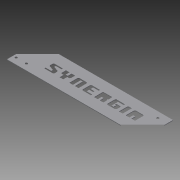
# Autodesk Inventor part: logo
Saved by Autodesk Inventor 2015 SP1 (Build 190203100, 203)
## iProperties
Created: 2015-04-17
Part Number: logo
Material: Ogólny
Document SubType Name: Konstrukcja blachowa
Designer: Marcin
Density: 1 g/cm^3
Appearance: Domyślna
Sheet Metal Rule: Domyślny
Author: Marcin
Autodesk Inventor part; units mm, degrees
ref_plane "YZ Plane" through (0, 0, 0) normal (1, 0, 0) x (0, 1, 0)
ref_plane "XZ Plane" through (0, 0, 0) normal (0, 1, 0) x (-1, 0, 0)
ref_plane "XY Plane" through (0, 0, 0) normal (0, 0, 1) x (1, 0, 0)
sketch "Szkic3" plane through (0, 0, 0) normal (0, 0, 1) x (1, 0, 0)
  line L0 (-89, -20) -> (89, -20)
  line L1 (89, -20) -> (89, 20)
  line L2 (89, 20) -> (-89, 20)
  line L3 (-89, 20) -> (-89, -20)
  line L4 (-89, -20) -> (89, 20) construction
  line L5 (89, -20) -> (-89, 20) construction
  point P0 (0, 0)
  dimension "d3" = 40
  dimension "d4" = 178
  measures "d3" distance of L0.end L1.end
  measures "d4" distance of L1.end L2.end
extrude "Płyta1" add sketch "Szkic3" along normal blind 0.8
sketch "Blok1" plane through (0, 0, 0) normal (0, 0, 1) x (1, 0, 0)
  line L0 (194.8054, -79.0716) -> (189.6563, -79.0716)
  line L1 (189.6563, -79.0716) -> (189.6563, -80.7591)
  line L2 (189.6563, -80.7591) -> (191.2238, -80.7591)
  line L3 (191.2238, -80.7591) -> (191.2238, -84.2418)
  line L4 (191.2238, -84.2418) -> (188.4658, -84.2418)
  line L5 (188.4658, -84.2418) -> (188.4658, -75.6126)
  line L6 (199.9976, -85.9056) -> (204.832, -85.9056)
  line L7 (204.832, -85.9056) -> (204.832, -73.9056)
  line L8 (204.832, -73.9056) -> (201.1445, -73.9056)
  line L9 (199.9976, -85.9056) -> (199.9976, -75.0767)
  line L10 (199.9976, -75.0767) -> (201.1445, -73.9056)
  line L11 (208.9177, -85.9056) -> (213.7175, -85.9056)
  line L12 (213.7175, -85.9056) -> (213.7175, -80.7591)
  line L13 (213.7175, -80.7591) -> (216.4159, -80.7591)
  line L14 (216.4159, -80.7591) -> (216.4159, -85.9056)
  line L15 (216.4159, -85.9056) -> (221.086, -85.9056)
  line L16 (221.086, -85.9056) -> (221.086, -75.0767)
  line L17 (221.086, -75.0767) -> (220.0494, -73.9056)
  line L18 (220.0494, -73.9056) -> (210.0722, -73.9056)
  line L19 (210.0722, -73.9056) -> (208.9177, -75.0767)
  line L20 (208.9177, -75.0767) -> (208.9177, -85.9056)
  line L21 (213.6195, -79.0716) -> (216.4159, -79.0716)
  line L22 (216.4159, -79.0716) -> (216.4159, -75.6126)
  line L23 (216.4159, -75.6126) -> (213.7175, -75.6126)
  line L24 (213.7175, -75.6126) -> (213.6195, -75.6126)
  line L25 (213.6195, -75.6126) -> (213.6195, -79.0716)
  line L26 (188.4658, -75.6126) -> (195.9066, -75.6126)
  line L27 (102.1862, -84.2418) -> (102.1862, -85.9056)
  line L28 (102.1862, -85.9056) -> (113.4232, -85.9056)
  line L29 (113.4232, -85.9056) -> (114.3485, -84.8496)
  line L30 (114.3485, -84.8496) -> (114.3485, -81.0367)
  line L31 (114.3485, -81.0367) -> (113.5668, -80.0795)
  line L32 (113.5668, -80.0795) -> (106.7866, -77.6387)
  line L33 (106.7866, -77.6387) -> (106.7866, -75.6126)
  line L34 (106.7866, -75.6126) -> (114.3485, -75.6126)
  line L35 (114.3485, -75.6126) -> (114.3485, -73.9056)
  line L36 (114.3485, -73.9056) -> (103.2928, -73.9056)
  line L37 (103.2928, -73.9056) -> (102.3186, -75.0175)
  line L38 (102.3186, -75.0175) -> (102.1862, -78.6916)
  line L39 (102.1862, -78.6916) -> (103.0668, -79.7699)
  line L40 (103.0668, -79.7699) -> (109.5514, -82.1043)
  line L41 (109.5514, -82.1043) -> (109.5514, -84.2418)
  line L42 (109.5514, -84.2418) -> (102.1862, -84.2418)
  line L43 (118.5153, -73.9056) -> (118.5153, -79.3691)
  line L44 (118.5153, -79.3691) -> (119.5796, -80.6723)
  line L45 (119.5796, -80.6723) -> (122.2512, -80.6723)
  line L46 (122.2512, -80.6723) -> (122.2512, -85.9056)
  line L47 (122.2512, -85.9056) -> (126.8723, -85.9056)
  line L48 (126.8723, -85.9056) -> (126.8723, -80.6723)
  line L49 (126.8723, -80.6723) -> (129.6451, -80.6723)
  line L50 (129.6451, -80.6723) -> (130.5602, -79.6279)
  line L51 (130.5602, -79.6279) -> (130.5602, -73.9056)
  line L52 (130.5602, -73.9056) -> (125.9666, -73.9056)
  line L53 (125.9666, -73.9056) -> (125.9666, -79.0339)
  line L54 (125.9666, -79.0339) -> (123.1426, -79.0339)
  line L55 (123.1426, -79.0339) -> (123.1426, -73.9056)
  line L56 (123.1426, -73.9056) -> (118.5153, -73.9056)
  line L57 (134.8965, -85.9056) -> (139.482, -85.9056)
  line L58 (139.482, -85.9056) -> (139.482, -75.6126)
  line L59 (139.482, -75.6126) -> (142.2406, -75.6126)
  line L60 (142.2406, -75.6126) -> (142.2406, -85.9056)
  line L61 (142.2406, -85.9056) -> (146.9336, -85.9056)
  line L62 (146.9336, -85.9056) -> (146.9336, -75.2319)
  line L63 (146.9336, -75.2319) -> (145.8504, -73.9056)
  line L64 (145.8504, -73.9056) -> (136.007, -73.9056)
  line L65 (136.007, -73.9056) -> (134.8965, -75.1731)
  line L66 (134.8965, -75.1731) -> (134.8965, -85.9056)
  line L67 (163.2215, -85.9056) -> (163.2215, -84.2418)
  line L68 (163.2215, -84.2418) -> (155.8113, -84.2418)
  line L69 (155.8113, -84.2418) -> (155.8113, -80.7591)
  line L70 (155.8113, -80.7591) -> (160.8725, -80.7591)
  line L71 (160.8725, -80.7591) -> (160.8725, -79.0339)
  line L72 (160.8725, -79.0339) -> (155.8113, -79.0339)
  line L73 (155.8113, -79.0339) -> (155.8113, -75.6126)
  line L74 (155.8113, -75.6126) -> (163.2215, -75.6126)
  line L75 (163.2215, -75.6126) -> (163.2215, -73.9056)
  line L76 (163.2215, -73.9056) -> (152.3241, -73.9056)
  line L77 (152.3241, -73.9056) -> (151.2136, -75.1731)
  line L78 (151.2136, -75.1731) -> (151.2136, -84.8496)
  line L79 (151.2136, -84.8496) -> (152.3241, -85.9056)
  line L80 (152.3241, -85.9056) -> (163.2215, -85.9056)
  line L81 (167.3998, -85.9056) -> (172.1189, -85.9056)
  line L82 (172.1189, -85.9056) -> (172.1189, -80.6723)
  line L83 (172.1189, -80.6723) -> (174.8793, -80.6723)
  line L84 (174.8793, -80.6723) -> (174.8793, -85.9056)
  line L85 (174.8793, -85.9056) -> (179.5438, -85.9056)
  line L86 (179.5438, -85.9056) -> (179.5438, -81.0367)
  line L87 (179.5438, -81.0367) -> (178.6965, -80.0795)
  line L88 (178.6965, -80.0795) -> (178.6965, -79.8231)
  line L89 (178.6965, -79.8231) -> (179.5438, -78.9321)
  line L90 (179.5438, -78.9321) -> (179.5438, -75.0767)
  line L91 (179.5438, -75.0767) -> (178.4192, -74.0073)
  line L92 (178.4192, -74.0073) -> (168.5273, -74.0834)
  line L93 (168.5273, -74.0834) -> (167.3998, -75.2692)
  line L94 (167.3998, -75.2692) -> (167.3998, -85.9056)
  line L95 (172.1189, -75.6126) -> (172.1189, -79.0339)
  line L96 (172.1189, -79.0339) -> (174.8793, -79.0339)
  line L97 (174.8793, -79.0339) -> (174.8793, -75.6126)
  line L98 (174.8793, -75.6126) -> (172.1189, -75.6126)
  line L99 (195.9066, -75.6126) -> (195.9066, -73.9056)
  line L100 (195.9066, -73.9056) -> (184.8247, -73.9056)
  line L101 (184.8247, -73.9056) -> (183.7111, -75.0767)
  line L102 (183.7111, -75.0767) -> (183.7111, -84.7811)
  line L103 (183.7111, -84.7811) -> (184.7064, -85.9056)
  line L104 (184.7064, -85.9056) -> (194.8054, -85.9056)
  line L105 (194.8054, -85.9056) -> (195.9066, -84.7811)
  line L106 (195.9066, -84.7811) -> (195.9066, -80.1501)
  line L107 (195.9066, -80.1501) -> (194.8054, -79.0716)
  point P0 (162.2151, -79.6004)
  dimension "d0" = 12
  measures "d0" distance between parallel lines of L36 L28
sketch "Szkic4" plane through (0, 0, 0.8) normal (0, 0, 1) x (1, 0, 0)
  line L0 (-89, -20) -> (-89, 20) projected
  line L1 (38.5569, 1.0581) -> (33.4078, 1.0581)
  line L2 (33.4078, 1.0581) -> (33.4078, -0.6294)
  line L3 (33.4078, -0.6294) -> (34.9753, -0.6294)
  line L4 (34.9753, -0.6294) -> (34.9753, -4.1121)
  line L5 (34.9753, -4.1121) -> (32.2172, -4.1121)
  line L6 (32.2172, -4.1121) -> (32.2172, 4.5171)
  line L7 (43.7491, -5.7759) -> (48.5835, -5.7759)
  line L8 (48.5835, -5.7759) -> (48.5835, 6.2241)
  line L9 (48.5835, 6.2241) -> (44.8959, 6.2241)
  line L10 (43.7491, -5.7759) -> (43.7491, 5.053)
  line L11 (43.7491, 5.053) -> (44.8959, 6.2241)
  line L12 (52.6692, -5.7759) -> (57.469, -5.7759)
  line L13 (57.469, -5.7759) -> (57.469, -0.6294)
  line L14 (57.469, -0.6294) -> (60.1673, -0.6294)
  line L15 (60.1673, -0.6294) -> (60.1673, -5.7759)
  line L16 (60.1673, -5.7759) -> (64.8375, -5.7759)
  line L17 (64.8375, -5.7759) -> (64.8375, 5.053)
  line L18 (64.8375, 5.053) -> (63.8009, 6.2241)
  line L19 (63.8009, 6.2241) -> (53.8237, 6.2241)
  line L20 (53.8237, 6.2241) -> (52.6692, 5.053)
  line L21 (52.6692, 5.053) -> (52.6692, -5.7759)
  line L22 (57.371, 1.0581) -> (60.1673, 1.0581)
  line L23 (60.1673, 1.0581) -> (60.1673, 4.5171)
  line L24 (60.1673, 4.5171) -> (57.469, 4.5171)
  line L25 (57.469, 4.5171) -> (57.371, 4.5171)
  line L26 (57.371, 4.5171) -> (57.371, 1.0581)
  line L27 (32.2172, 4.5171) -> (39.6581, 4.5171)
  line L28 (-54.0623, -4.1121) -> (-54.0623, -5.7759)
  line L29 (-54.0623, -5.7759) -> (-42.8254, -5.7759)
  line L30 (-42.8254, -5.7759) -> (-41.9001, -4.7199)
  line L31 (-41.9001, -4.7199) -> (-41.9001, -0.9071)
  line L32 (-41.9001, -0.9071) -> (-42.6818, 0.0501)
  line L33 (-42.6818, 0.0501) -> (-49.4619, 2.491)
  line L34 (-49.4619, 2.491) -> (-49.4619, 4.5171)
  line L35 (-49.4619, 4.5171) -> (-41.9001, 4.5171)
  line L36 (-41.9001, 4.5171) -> (-41.9001, 6.2241)
  line L37 (-41.9001, 6.2241) -> (-52.9557, 6.2241)
  line L38 (-52.9557, 6.2241) -> (-53.9299, 5.1122)
  line L39 (-53.9299, 5.1122) -> (-54.0623, 1.4381)
  line L40 (-54.0623, 1.4381) -> (-53.1817, 0.3598)
  line L41 (-53.1817, 0.3598) -> (-46.6971, -1.9747)
  line L42 (-46.6971, -1.9747) -> (-46.6971, -4.1121)
  line L43 (-46.6971, -4.1121) -> (-54.0623, -4.1121)
  line L44 (-37.7332, 6.2241) -> (-37.7332, 0.7606)
  line L45 (-37.7332, 0.7606) -> (-36.6689, -0.5426)
  line L46 (-36.6689, -0.5426) -> (-33.9974, -0.5426)
  line L47 (-33.9974, -0.5426) -> (-33.9974, -5.7759)
  line L48 (-33.9974, -5.7759) -> (-29.3763, -5.7759)
  line L49 (-29.3763, -5.7759) -> (-29.3763, -0.5426)
  line L50 (-29.3763, -0.5426) -> (-26.6034, -0.5426)
  line L51 (-26.6034, -0.5426) -> (-25.6884, 0.5017)
  line L52 (-25.6884, 0.5017) -> (-25.6884, 6.2241)
  line L53 (-25.6884, 6.2241) -> (-30.282, 6.2241)
  line L54 (-30.282, 6.2241) -> (-30.282, 1.0958)
  line L55 (-30.282, 1.0958) -> (-33.1059, 1.0958)
  line L56 (-33.1059, 1.0958) -> (-33.1059, 6.2241)
  line L57 (-33.1059, 6.2241) -> (-37.7332, 6.2241)
  line L58 (-21.3521, -5.7759) -> (-16.7665, -5.7759)
  line L59 (-16.7665, -5.7759) -> (-16.7665, 4.5171)
  line L60 (-16.7665, 4.5171) -> (-14.008, 4.5171)
  line L61 (-14.008, 4.5171) -> (-14.008, -5.7759)
  line L62 (-14.008, -5.7759) -> (-9.3149, -5.7759)
  line L63 (-9.3149, -5.7759) -> (-9.3149, 4.8978)
  line L64 (-9.3149, 4.8978) -> (-10.3981, 6.2241)
  line L65 (-10.3981, 6.2241) -> (-20.2415, 6.2241)
  line L66 (-20.2415, 6.2241) -> (-21.3521, 4.9566)
  line L67 (-21.3521, 4.9566) -> (-21.3521, -5.7759)
  line L68 (6.9729, -5.7759) -> (6.9729, -4.1121)
  line L69 (6.9729, -4.1121) -> (-0.4373, -4.1121)
  line L70 (-0.4373, -4.1121) -> (-0.4373, -0.6294)
  line L71 (-0.4373, -0.6294) -> (4.624, -0.6294)
  line L72 (4.624, -0.6294) -> (4.624, 1.0958)
  line L73 (4.624, 1.0958) -> (-0.4373, 1.0958)
  line L74 (-0.4373, 1.0958) -> (-0.4373, 4.5171)
  line L75 (-0.4373, 4.5171) -> (6.9729, 4.5171)
  line L76 (6.9729, 4.5171) -> (6.9729, 6.2241)
  line L77 (6.9729, 6.2241) -> (-3.9244, 6.2241)
  line L78 (-3.9244, 6.2241) -> (-5.035, 4.9566)
  line L79 (-5.035, 4.9566) -> (-5.035, -4.7199)
  line L80 (-5.035, -4.7199) -> (-3.9244, -5.7759)
  line L81 (-3.9244, -5.7759) -> (6.9729, -5.7759)
  line L82 (11.1513, -5.7759) -> (15.8704, -5.7759)
  line L83 (15.8704, -5.7759) -> (15.8704, -0.5426)
  line L84 (15.8704, -0.5426) -> (18.6308, -0.5426)
  line L85 (18.6308, -0.5426) -> (18.6308, -5.7759)
  line L86 (18.6308, -5.7759) -> (23.2953, -5.7759)
  line L87 (23.2953, -5.7759) -> (23.2953, -0.9071)
  line L88 (23.2953, -0.9071) -> (22.448, 0.0501)
  line L89 (22.448, 0.0501) -> (22.448, 0.3065)
  line L90 (22.448, 0.3065) -> (23.2953, 1.1975)
  line L91 (23.2953, 1.1975) -> (23.2953, 5.053)
  line L92 (23.2953, 5.053) -> (22.1707, 6.1224)
  line L93 (22.1707, 6.1224) -> (12.2788, 6.0462)
  line L94 (12.2788, 6.0462) -> (11.1513, 4.8605)
  line L95 (11.1513, 4.8605) -> (11.1513, -5.7759)
  line L96 (15.8704, 4.5171) -> (15.8704, 1.0958)
  line L97 (15.8704, 1.0958) -> (18.6308, 1.0958)
  line L98 (18.6308, 1.0958) -> (18.6308, 4.5171)
  line L99 (18.6308, 4.5171) -> (15.8704, 4.5171)
  line L100 (39.6581, 4.5171) -> (39.6581, 6.2241)
  line L101 (39.6581, 6.2241) -> (28.5761, 6.2241)
  line L102 (28.5761, 6.2241) -> (27.4626, 5.053)
  line L103 (27.4626, 5.053) -> (27.4626, -4.6515)
  line L104 (27.4626, -4.6515) -> (28.4579, -5.7759)
  line L105 (28.4579, -5.7759) -> (38.5569, -5.7759)
  line L106 (38.5569, -5.7759) -> (39.6581, -4.6515)
  line L107 (39.6581, -4.6515) -> (39.6581, -0.0204)
  line L108 (39.6581, -0.0204) -> (38.5569, 1.0581)
  point P0 (0, 0)
extrude "Wytnij1" cut sketch "Szkic4" against normal blind 0.8 contours L108 L107 L106 L105 L104 L103 L102 L101 L100 L27 L6 L5 L4 L3 L2 L1 | L10 L11 L9 L8 L7 | L21 L20 L19 L18 L17 L16 L15 L14 L13 L12 | L26 L25 L24 L23 L22 | L43 L42 L41 L40 L39 L38 L37 L36 L35 L34 L33 L32 L31 L30 L29 L28 | L57 L56 L55 L54 L53 L52 L51 L50 L49 L48 L47 L46 L45 L44 | L67 L66 L65 L64 L63 L62 L61 L60 L59 L58 | L81 L80 L79 L78 L77 L76 L75 L74 L73 L72 L71 L70 L69 L68 | L95 L94 L93 L92 L91 L90 L89 L88 L87 L86 L85 L84 L83 L82 | L99 L98 L97 L96
sketch "Szkic7" plane through (0, 0, 0.8) normal (0, 0, 1) x (1, 0, 0)
  circle A0 centre (-84.9, -12) radius 1.5 projected
  circle A1 centre (-71.4, -12) radius 1.5 projected
  circle A2 centre (-71.4, 12) radius 1.5 projected
  circle A3 centre (-84.9, 12) radius 1.5 projected
  point P0 (0, 0)
  constraints: 4 coincident
hole "Otwór1" at (-84.9, -12, 0.8) at (-71.4, -12, 0.8) at (-71.4, 12, 0.8) at (-84.9, 12, 0.8) direction (0, 0, -1) diameter 3 depth 0.8 tip angle 118
sketch "Szkic8" plane through (0, 0, 0.8) normal (0, 0, 1) x (1, 0, 0)
  circle A0 centre (-71.4, -12) radius 1.5 projected
  circle A1 centre (-71.4, 12) radius 1.5 projected
  line L0 (-71.4, 12) -> (115.8651, 12) construction
  line L1 (-89, 20) -> (-89, -20) construction
  line L2 (-89, 0) -> (89, 0) construction
  line L3 (89, -20) -> (89, 20) construction
  line L4 (77, 12) -> (77, -12) construction
  point P0 (0, 0)
  dimension "d35" = 12
  constraints: 6 end point, 2 midpoint, 1 coincident, 1 horizontal, 1 point on line, 1 symmetric about line, 1 vertical
  measures "d35" distance from line of L3 L4.start
hole "Otwór2" at (77, 12, 0.8) at (77, -12, 0.8) direction (0, 0, -1) diameter 3 depth 0.8 tip angle 118
equation "\"d6\" = Grubość"
equation "\"d33\" = Grubość"
equation "\"d41\" = Grubość"
equation "\"PromieńGięcia\" = Grubość"
equation "\"SzerokośćGięciaPodcięcia\" = Grubość"
equation "\"GłębokośćGięciaPodcięcia\" = 0.5 * Grubość"
equation "\"RozmiarPodcięciaNarożnika\" = 4 * Grubość"
equation "\"MinimalnaPozostałość\" = 2 * Grubość"
equation "\"PromieńPrzejścia\" = PromieńGięcia"
equation "\"Rozmiar_promienia_Jacobiego\" = Grubość"
equation "\"Wielk_odstępu\" = Grubość"
equation "\"d5\" = PromieńGięcia"
equation "\"Grubość\" = 0.8"
